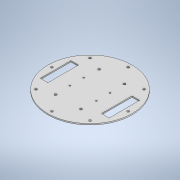
# Autodesk Inventor part: pcbCase
Saved by Autodesk Inventor 2020 (Build 240168000, 168)
## iProperties
Created: 2020-04-07
Part Number: pcbCase
Material: Типовые
Document SubType Name: Modeling
Designer: jamnissa
Density: 1 g/cm^3
Appearance: По умолчанию
Author: jamnissa
Autodesk Inventor part; units mm, degrees
ref_plane "YZ Plane" through (0, 0, 0) normal (1, 0, 0) x (0, 1, 0)
ref_plane "XZ Plane" through (0, 0, 0) normal (0, 1, 0) x (-1, 0, 0)
ref_plane "XY Plane" through (0, 0, 0) normal (0, 0, 1) x (1, 0, 0)
sketch "Эскиз1" plane through (0, 0, 0) normal (0, 1, 0) x (-1, 0, 0)
  circle A0 centre (0, 0) radius 55
  line L0 (79.4555, 0) -> (-79.4555, 0)
  line L1 (0, -103.8803) -> (0, 88.3129)
  dimension "d0" = 110
  constraints: 4 end point, 1 centre point, 1 coincident, 1 horizontal, 1 midpoint, 1 point on line, 1 vertical
  measures "d0" diameter of A0
extrude "Выдавливание1" add sketch "Эскиз1" along normal blind 1.6
sketch "Эскиз2" plane through (0, 0, 0) normal (0, -1, 0) x (1, 0, 0)
  circle A0 centre (0, 0) radius 55 projected
  line L0 (0, -103.8803) -> (0, 88.3129) projected
  line L1 (-79.4555, 0) -> (79.4555, 0) projected
  line L2 (11.5, -13.3) -> (23, -13.3)
  line L3 (23, -13.3) -> (23, 13.3)
  line L4 (23, 13.3) -> (11.5, 13.3)
  line L5 (11.5, 13.3) -> (11.5, -13.3)
  line L6 (35, -20) -> (45, -20)
  line L7 (45, -20) -> (45, 20)
  line L8 (45, 20) -> (35, 20)
  line L9 (35, 20) -> (35, -20)
  line L10 (17.25, -13.3) -> (17.25, 13.3)
  circle A1 centre (17.25, -9) radius 1
  circle A2 centre (17.25, 9) radius 1
  line L11 (3, 6) -> (33, 6)
  line L12 (33, 6) -> (33, -6)
  line L13 (33, -6) -> (3, -6)
  line L14 (3, -6) -> (3, 6)
  line L15 (-11.5, -13.3) -> (-23, -13.3)
  line L16 (-23, -13.3) -> (-23, 13.3)
  line L17 (-23, 13.3) -> (-11.5, 13.3)
  line L18 (-11.5, 13.3) -> (-11.5, -13.3)
  line L19 (-35, -20) -> (-45, -20)
  line L20 (-45, -20) -> (-45, 20)
  line L21 (-45, 20) -> (-35, 20)
  line L22 (-35, 20) -> (-35, -20)
  line L23 (-17.25, -13.3) -> (-17.25, 13.3)
  circle A3 centre (-17.25, -9) radius 1
  circle A4 centre (-17.25, 9) radius 1
  line L24 (-3, 6) -> (-33, 6)
  line L25 (-33, 6) -> (-33, -6)
  line L26 (-33, -6) -> (-3, -6)
  line L27 (-3, -6) -> (-3, 6)
  circle A5 centre (0, 0) radius 50
  circle A6 centre (0, -50) radius 1.5
  circle A7 centre (50, 0) radius 1.5
  circle A8 centre (0, 50) radius 1.5
  circle A9 centre (-50, 0) radius 1.5
  circle A10 centre (35.3553, -35.3553) radius 1.5
  circle A11 centre (50, 0) radius 1.5
  circle A12 centre (35.3553, 35.3553) radius 1.5
  circle A13 centre (0, 50) radius 1.5
  circle A14 centre (-35.3553, 35.3553) radius 1.5
  circle A15 centre (-50, 0) radius 1.5
  circle A16 centre (-35.3553, -35.3553) radius 1.5
  dimension "d6" = 11.5
  dimension "d7" = 26.6
  dimension "d9" = 10
  dimension "d10" = 40
  dimension "d11" = 45
  dimension "d12" = 12
  dimension "d13" = 2
  dimension "d14" = 18
  dimension "d15" = 2
  dimension "d16" = 30
  dimension "d17" = 12
  dimension "d18" = 2
  dimension "d21" = 100
  dimension "d22" = 3
  dimension "d23" = 3
  dimension "d25" = 3
  dimension "d26" = 3
  dimension "d30" = 360
  constraints: 52 end point, 17 symmetric about line, 16 centre point, 8 point on line, 6 parallel, 4 point on circle, 3 horizontal, 3 perpendicular, 2 midpoint, 1 coincident, 22 other
  measures "d6" distance of L3.end L4.end
  measures "d7" distance of L2.end L3.end
  measures "d9" distance of L8.end L7.end
  measures "d10" distance of L8.end L6.start
  measures "d11" distance from line of L7 A0.centre
  measures "d12" distance between parallel lines of L9 L3
  measures "d13" diameter of A2
  measures "d14" distance of A2.centre A1.centre
  measures "d15" diameter of A1
  measures "d16" distance of L13.end L12.end
  measures "d17" distance of L13.end L11.start
  measures "d18" distance between parallel lines of L9 L12
  measures "d21" diameter of A5
  measures "d22" diameter of A6
  measures "d23" diameter of A7
  measures "d25" diameter of A8
  measures "d26" diameter of A9
extrude "Выдавливание2" cut sketch "Эскиз2" against normal blind 1.6 contours A7 A5 L1 | L1 A5 A7 | A8 A5 L0 | L0 A5 A8 | A6 A5 L0 | L0 A5 A6 | A5 A7 L1 | L1 A7 A5 | A9 A5 L1 | L1 A5 A9 | A5 A8 L0 | L0 A8 A5 | A5 A6 L0 | L0 A6 A5 | A12 A5 | A5 A12 | A10 A5 | A5 A10 | A5 A9 L1 | L1 A9 A5 | A14 A5 | A5 A14 | A16 A5 | A5 A16 | L7 L6 L9 L1 | L1 L9 L8 L7 | L20 L21 L22 L1 | L1 L22 L19 L20 | A3 L23 | L23 A3 | A4 L23 | L23 A4 | A1 L10 | L10 A1 | A2 L10 | L10 A2
sketch "Эскиз3" plane through (0, 0, 0) normal (0, -1, 0) x (1, 0, 0)
  circle A0 centre (50, 0) radius 1.5 projected
  circle A1 centre (-50, 0) radius 1.5 projected
  circle A2 centre (-17.25, 9) radius 1 projected
  line L0 (35, -20) -> (35, 20) projected
  line L1 (35, 20) -> (45, 20) projected
  line L2 (45, 20) -> (45, -20) projected
  line L3 (45, -20) -> (35, -20) projected
  line L4 (-35, -20) -> (-45, -20) projected
  line L5 (-45, -20) -> (-45, 20) projected
  line L6 (-45, 20) -> (-35, 20) projected
  line L7 (-35, 20) -> (-35, -20) projected
  circle A3 centre (-35.3553, 35.3553) radius 1.5 projected
  circle A4 centre (35.3553, -35.3553) radius 1.5 projected
  circle A5 centre (35.3553, 35.3553) radius 1.5 projected
  circle A6 centre (-35.3553, -35.3553) radius 1.5 projected
  circle A7 centre (17.25, 9) radius 1 projected
  circle A8 centre (17.25, -9) radius 1 projected
  circle A9 centre (-17.25, -9) radius 1 projected
  circle A10 centre (0, 50) radius 1.5 projected
  circle A11 centre (0, -50) radius 1.5 projected
  circle A12 centre (0, 0) radius 55 projected
  line L8 (-79.4555, 0) -> (79.4555, 0) projected
  line L9 (0, -103.8803) -> (0, 88.3129) projected
  circle A13 centre (0, 0) radius 50 projected
  circle A14 centre (-35.3553, -35.3553) radius 1.5 projected
  line L10 (23, 13.3) -> (11.5, 13.3) projected
  line L11 (-21.1, -39.0646) -> (21.1, -39.0646)
  line L12 (21.1, -39.0646) -> (21.1, 37.2354)
  line L13 (21.1, 37.2354) -> (-21.1, 37.2354)
  line L14 (-21.1, 37.2354) -> (-21.1, -39.0646)
  circle A15 centre (-16.5, -28.5) radius 1.5
  circle A16 centre (16.5, -28.5) radius 1.5
  circle A17 centre (16.5, 28.5) radius 1.5
  circle A18 centre (-16.5, 28.5) radius 1.5
  dimension "d34" = 76.3
  dimension "d35" = 42.2
  dimension "d37" = 3
  dimension "d38" = 3
  dimension "d39" = 3
  dimension "d40" = 3
  dimension "d42" = 33
  dimension "d43" = 57
  constraints: 8 end point, 4 centre point, 3 symmetric about line, 2 parallel, 1 horizontal, 1 perpendicular, 1 other
  measures "d34" distance of L11.end L12.end
  measures "d35" distance of L12.end L13.end
  measures "d37" diameter of A15
  measures "d38" diameter of A16
  measures "d39" diameter of A17
  measures "d40" diameter of A18
  measures "d42" distance of A17.centre A18.centre
  measures "d43" distance of A18.centre A15.centre
extrude "Выдавливание3" cut sketch "Эскиз3" against normal blind 1.6 contours A15 | A16 | A17 | A18
